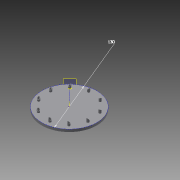
# Autodesk Inventor part: inner bayonet connector 10
Saved by Autodesk Inventor 2015 (Build 190159000, 159)
## iProperties
Created: 2014-09-30
Part Number: inner bayonet connector 10
Material: Generic
Document SubType Name: Modeling
Designer: ericd_000
Density: 1 g/cm^3
Appearance: Default
Author: ericd_000
Autodesk Inventor part; units mm, degrees
ref_plane "YZ Plane" through (0, 0, 0) normal (1, 0, 0) x (0, 1, 0)
ref_plane "XZ Plane" through (0, 0, 0) normal (0, 1, 0) x (-1, 0, 0)
ref_plane "XY Plane" through (0, 0, 0) normal (0, 0, 1) x (1, 0, 0)
sketch "Sketch14" plane through (0, 0, 0) normal (0, 0, 1) x (1, 0, 0)
  circle A0 centre (0, 0) radius 65
  dimension "d67" = 130
  constraints: 1 centre point, 1 coincident
  measures "d67" diameter of A0
extrude "Extrusion10" add sketch "Sketch14" along normal blind 6
sketch "Sketch15" plane through (0, 0, 6) normal (0, 0, 1) x (1, 0, 0)
  circle A0 centre (-37.7323, 38.6299) radius 2
  line L0 (-37.7323, 38.6299) -> (0, 0) construction
  circle A1 centre (0, 0) radius 65 projected
  line L1 (0, 0) -> (-55.3564, 56.6733) construction
  line L2 (-55.3564, 56.6733) -> (-63.1164, 49.0935) construction
  dimension "d70" = 54
  dimension "d75" = 4
  constraints: 6 end point, 1 centre point, 1 perpendicular
  measures "d70" distance of L0.start L0.end
  measures "d75" diameter of A0
extrude "Extrusion11" cut sketch "Sketch15" against normal blind 6 contours A0
sketch "Sketch16" plane through (0, 0, 6) normal (0, 0, 1) x (1, 0, 0)
  circle A0 centre (-37.7323, 38.6299) radius 2.75
  circle A1 centre (-37.7323, 38.6299) radius 2 projected
  point P0 (0, 0)
  dimension "d73" = 5.5
  constraints: 1 centre point, 1 concentric
  measures "d73" diameter of A0
extrude "Extrusion12" add sketch "Sketch16" along normal blind 8
sketch "Sketch17" plane through (0, 0, 6) normal (0, 0, 1) x (1, 0, 0)
  circle A0 centre (-37.7323, 38.6299) radius 2.75 projected
  circle A1 centre (-37.7323, 38.6299) radius 2 construction
  line L0 (-37.7323, 38.6299) -> (0, 0) construction
  line L1 (-37.7323, 38.6299) -> (-45.4185, 46.499) construction
  circle A2 centre (0, 0) radius 65 construction
  dimension "d79" = 130
  constraints: 4 end point, 1 coincident, 1 collinear, 3 other
ref_plane "Work Plane18" through (-45.4185, 46.499, 6) normal (-0.6987, 0.7154, 0) x (-0.7154, -0.6987, 0)
sketch "Sketch18" plane through (-45.4185, 46.499, 6) normal (-0.6987, 0.7154, 0) x (-0.7154, -0.6987, 0)
  line L0 (-2.7631, 8) -> (2.8739, 3.2761)
  line L1 (2.8739, 3.2761) -> (2.8739, 8)
  line L2 (2.8739, 8) -> (-2.7631, 8)
  point P0 (0, -6)
  constraints: 6 end point, 1 horizontal, 1 vertical
extrude "Extrusion13" cut sketch "Sketch18" against normal blind 15
pattern_circular "Circular Pattern2" count 10 over 360 about axis through (0, 0, 6) along (0, 0, 1) of "Extrusion12", "Extrusion13", "Extrusion11"
body "Solid2"
